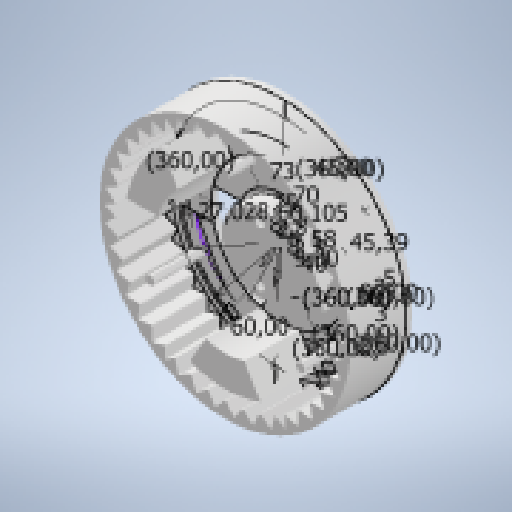
# Autodesk Inventor part: wheel_mold
Saved by Autodesk Inventor 2023 (Build 270158000, 158)
## iProperties
Created: 2026-02-22
Part Number: wheel_mold
Material: Типовые
Document SubType Name: Modeling
Designer: garin
Density: 1 g/cm^3
Appearance: По умолчанию
Author: garin
Autodesk Inventor part; units mm, degrees
ref_plane "YZ Plane" through (0, 0, 0) normal (1, 0, 0) x (0, 1, 0)
ref_plane "XZ Plane" through (0, 0, 0) normal (0, 1, 0) x (-1, 0, 0)
sketch "Эскиз1" plane through (0, 0, 0) normal (0, 0, 1) x (1, 0, 0)
  circle A0 centre (0, 0) radius 35
  circle A1 centre (0, 0) radius 20
  line L0 (0, 0) -> (34.569092, 5.475206) construction
  line L1 (0, 0) -> (35, 0) construction
  line L2 (0, 0) -> (34.569092, -5.475206) construction
  line L3 (34.569092, 5.475206) -> (29.63065, 4.693034) construction
  line L4 (29.63065, 4.693034) -> (19.44159, 4.693034) construction
  line L5 (19.44159, 4.693034) -> (34.683936, 4.693034)
  line L6 (19.44159, -4.693034) -> (34.683936, -4.693034)
  line L7 (13.785082, 14.490394) -> (21.406255, 27.690653) construction
  line L8 (10.751038, 28.007413) -> (5.656509, 19.183428) construction
  line L9 (5.656509, 19.183428) -> (13.277681, 32.383687) construction
  line L10 (-5.656509, 19.183428) -> (-13.277681, 32.383687) construction
  line L11 (-18.879612, 23.314379) -> (-13.785082, 14.490394) construction
  line L12 (-13.785082, 14.490394) -> (-21.406255, 27.690653)
  line L13 (-19.44159, 4.693034) -> (-34.683936, 4.693034)
  line L14 (-29.63065, -4.693034) -> (-19.44159, -4.693034) construction
  line L15 (-19.44159, -4.693034) -> (-34.683936, -4.693034) construction
  line L16 (-13.785082, -14.490394) -> (-21.406255, -27.690653) construction
  line L17 (-10.751038, -28.007413) -> (-5.656509, -19.183428) construction
  line L18 (-5.656509, -19.183428) -> (-13.277681, -32.383687)
  line L19 (5.656509, -19.183428) -> (13.277681, -32.383687) construction
  line L20 (18.879612, -23.314379) -> (13.785082, -14.490394) construction
  line L21 (13.785082, -14.490394) -> (21.406255, -27.690653) construction
  line L22 (0, 0) -> (17.5, 30.310889) construction
  line L23 (0, 0) -> (-17.5, 30.310889) construction
  line L24 (0, 0) -> (-35, 0) construction
  line L25 (0, 0) -> (-17.5, -30.310889) construction
  line L26 (0, 0) -> (17.5, -30.310889) construction
  line L27 (34.683936, 4.693034) -> (29.683936, 4.693034) construction
  line L28 (29.683936, 4.693034) -> (29.683936, -4.693034)
  line L29 (29.683936, 4.693034) -> (29.683936, 1.693034)
  line L30 (29.683936, 1.693034) -> (34.959028, 1.693034)
  line L31 (29.683936, -4.693034) -> (29.683936, -1.693034) construction
  line L32 (29.683936, -1.693034) -> (34.959028, -1.693034)
  line L33 (13.785082, 14.490394) -> (21.406255, 27.690653)
  line L34 (10.751038, 28.007413) -> (5.656509, 19.183428)
  line L35 (13.375758, 26.55356) -> (16.013304, 31.121923)
  line L36 (5.656509, 19.183428) -> (13.277681, 32.383687) construction
  line L37 (10.777681, 28.05356) -> (18.906255, 23.360526)
  line L38 (16.308179, 24.860526) -> (18.945724, 29.428889)
  line L39 (-5.656509, 19.183428) -> (-13.277681, 32.383687) construction
  line L40 (-18.879612, 23.314379) -> (-13.785082, 14.490394)
  line L41 (-16.308179, 24.860526) -> (-18.945724, 29.428889)
  line L42 (-13.785082, 14.490394) -> (-21.406255, 27.690653) construction
  line L43 (-18.906255, 23.360526) -> (-10.777681, 28.05356)
  line L44 (-13.375758, 26.55356) -> (-16.013304, 31.121923)
  line L45 (-19.44159, 4.693034) -> (-34.683936, 4.693034) construction
  line L46 (-29.63065, -4.693034) -> (-19.44159, -4.693034)
  line L47 (-29.683936, -1.693034) -> (-34.959028, -1.693034)
  line L48 (-19.44159, -4.693034) -> (-34.683936, -4.693034) construction
  line L49 (-29.683936, -4.693034) -> (-29.683936, 4.693034)
  line L50 (-29.683936, 1.693034) -> (-34.959028, 1.693034)
  line L51 (-13.785082, -14.490394) -> (-21.406255, -27.690653) construction
  line L52 (-10.751038, -28.007413) -> (-5.656509, -19.183428)
  line L53 (-13.375758, -26.55356) -> (-16.013304, -31.121923)
  line L54 (-5.656509, -19.183428) -> (-13.277681, -32.383687) construction
  line L55 (-10.777681, -28.05356) -> (-18.906255, -23.360526)
  line L56 (-16.308179, -24.860526) -> (-18.945724, -29.428889)
  line L57 (5.656509, -19.183428) -> (13.277681, -32.383687)
  line L58 (18.879612, -23.314379) -> (13.785082, -14.490394)
  line L59 (16.308179, -24.860526) -> (18.945724, -29.428889)
  line L60 (13.785082, -14.490394) -> (21.406255, -27.690653) construction
  line L61 (18.906255, -23.360526) -> (10.777681, -28.05356)
  line L62 (13.375758, -26.55356) -> (16.013304, -31.121923)
  circle A2 centre (0, 0) radius 30.0525
  line L63 (21.406255, 27.690653) -> (20.197155, 25.596431) construction
  line L64 (18.945724, 29.428889) -> (17.445724, 26.830813) construction
  line L65 (17.445724, 26.830813) -> (21.211762, 27.83992)
  line L66 (0, 0) -> (21.211762, 27.83992) construction
  line L67 (21.238374, 23.941121) -> (21.211762, 27.83992)
  line L68 (24.749898, 20.290106) -> (25.338794, 24.144264)
  line L69 (21.46071, 23.742025) -> (25.338794, 24.144264)
  line L70 (27.641356, 16.130756) -> (28.831007, 19.843716)
  line L71 (24.938034, 20.058422) -> (28.831007, 19.843716)
  line L72 (29.840307, 11.567278) -> (31.600908, 15.046017)
  line L73 (27.790578, 15.87229) -> (31.600908, 15.046017)
  line L74 (31.29166, 6.714002) -> (33.579103, 9.871366)
  line L75 (29.946878, 11.288504) -> (33.579103, 9.871366)
  line L76 (31.959055, 1.692518) -> (34.716031, 4.449405)
  line L77 (31.35291, 6.421905) -> (34.716031, 4.449405)
  circle A3 centre (0, 0) radius 32.003841
  line L78 (-14.513304, 28.523847) -> (-13.504197, 32.289885)
  line L79 (-10.114432, 30.363532) -> (-13.504197, 32.289885)
  line L80 (-9.830842, 30.456532) -> (-8.240149, 34.016172)
  line L81 (-5.196798, 31.579093) -> (-8.240149, 34.016172)
  line L82 (14.513764, 28.523613) -> (13.504718, 32.289667)
  line L83 (10.114922, 30.363369) -> (13.504718, 32.289667)
  line L84 (9.831334, 30.456374) -> (8.240698, 34.016039)
  line L85 (5.197307, 31.579009) -> (8.240698, 34.016039)
  line L86 (4.902597, 31.626103) -> (2.770221, 34.890197)
  line L87 (0.149483, 32.003492) -> (2.770221, 34.890197)
  line L88 (-0.148967, 32.003494) -> (-2.769658, 34.890242)
  line L89 (-4.902086, 31.626182) -> (-2.769658, 34.890242)
  line L90 (-31.959028, 1.693034) -> (-34.715959, 4.449965)
  line L91 (-31.352806, 6.422411) -> (-34.715959, 4.449965)
  line L92 (-31.291552, 6.714507) -> (-33.578943, 9.871908)
  line L93 (-29.946696, 11.288988) -> (-33.578943, 9.871908)
  line L94 (-17.445291, 26.831095) -> (-21.211313, 27.840262)
  line L95 (-21.237988, 23.941464) -> (-21.211313, 27.840262)
  line L96 (-21.460327, 23.742372) -> (-25.338405, 24.144673)
  line L97 (-24.749571, 20.290505) -> (-25.338405, 24.144673)
  line L98 (-24.93771, 20.058825) -> (-28.830687, 19.844181)
  line L99 (-27.641095, 16.131202) -> (-28.830687, 19.844181)
  line L100 (-27.790322, 15.872738) -> (-31.600665, 15.046527)
  line L101 (-29.84012, 11.56776) -> (-31.600665, 15.046527)
  line L102 (-17.445724, -26.830813) -> (-21.211762, -27.83992)
  line L103 (-21.238374, -23.941121) -> (-21.211762, -27.83992)
  line L104 (-21.46071, -23.742025) -> (-25.338794, -24.144264)
  line L105 (-24.749898, -20.290106) -> (-25.338794, -24.144264)
  line L106 (-31.959055, -1.692518) -> (-34.716031, -4.449405)
  line L107 (-31.35291, -6.421905) -> (-34.716031, -4.449405)
  line L108 (-31.29166, -6.714002) -> (-33.579103, -9.871366)
  line L109 (-29.946878, -11.288504) -> (-33.579103, -9.871366)
  line L110 (-29.840307, -11.567278) -> (-31.600908, -15.046017)
  line L111 (-27.790578, -15.87229) -> (-31.600908, -15.046017)
  line L112 (-27.641356, -16.130756) -> (-28.831007, -19.843716)
  line L113 (-24.938034, -20.058422) -> (-28.831007, -19.843716)
  line L114 (14.513304, -28.523847) -> (13.504197, -32.289885)
  line L115 (10.114432, -30.363532) -> (13.504197, -32.289885)
  line L116 (9.830842, -30.456532) -> (8.240149, -34.016172)
  line L117 (5.196798, -31.579093) -> (8.240149, -34.016172)
  line L118 (-14.513764, -28.523613) -> (-13.504718, -32.289667)
  line L119 (-10.114922, -30.363369) -> (-13.504718, -32.289667)
  line L120 (-9.831334, -30.456374) -> (-8.240698, -34.016039)
  line L121 (-5.197307, -31.579009) -> (-8.240698, -34.016039)
  line L122 (-4.902597, -31.626103) -> (-2.770221, -34.890197)
  line L123 (-0.149483, -32.003492) -> (-2.770221, -34.890197)
  line L124 (0.148967, -32.003494) -> (2.769658, -34.890242)
  line L125 (4.902086, -31.626182) -> (2.769658, -34.890242)
  line L126 (31.959028, -1.693034) -> (34.715959, -4.449965)
  line L127 (31.352806, -6.422411) -> (34.715959, -4.449965)
  line L128 (31.291552, -6.714507) -> (33.578943, -9.871908)
  line L129 (29.946696, -11.288988) -> (33.578943, -9.871908)
  line L130 (17.445291, -26.831095) -> (21.211313, -27.840262)
  line L131 (21.237988, -23.941464) -> (21.211313, -27.840262)
  line L132 (21.460327, -23.742372) -> (25.338405, -24.144673)
  line L133 (24.749571, -20.290505) -> (25.338405, -24.144673)
  line L134 (24.93771, -20.058825) -> (28.830687, -19.844181)
  line L135 (27.641095, -16.131202) -> (28.830687, -19.844181)
  line L136 (27.790322, -15.872738) -> (31.600665, -15.046527)
  line L137 (29.84012, -11.56776) -> (31.600665, -15.046527)
  circle A4 centre (0, 0) radius 11
  line L138 (0, 0) -> (0, 8) construction
  circle A5 centre (0, 8) radius 1.25
  circle A6 centre (0, -8) radius 1.25
  line L139 (0, 0) -> (8, 0) construction
  circle A7 centre (8, 0) radius 1.25
  circle A8 centre (-8, 0) radius 1.25
  circle A9 centre (0, 0) radius 12.5
  circle A10 centre (0, 0) radius 36.5
  arc A11 (-13.785082, 14.490394) -> (-19.44159, 4.693034) centre (0, 0) ccw
  line L140 (-26.974922, 1.693034) -> (-26.974922, -1.693034)
  line L141 (-29.683936, 1.693034) -> (-26.974922, 1.693034)
  line L142 (-26.974922, -1.693034) -> (-29.683936, -1.693034)
  line L143 (-12.021251, -24.207485) -> (-13.375758, -26.55356)
  line L144 (-16.308179, -24.860526) -> (-14.953671, -22.514451)
  line L145 (-14.953671, -22.514451) -> (-12.021251, -24.207485)
  line L146 (14.953671, -22.514451) -> (16.308179, -24.860526)
  line L147 (13.375758, -26.55356) -> (12.021251, -24.207485)
  line L148 (12.021251, -24.207485) -> (14.953671, -22.514451)
  line L149 (26.974922, 1.693034) -> (29.683936, 1.693034)
  line L150 (29.683936, -1.693034) -> (26.974922, -1.693034)
  line L151 (26.974922, -1.693034) -> (26.974922, 1.693034)
  line L152 (12.021251, 24.207485) -> (13.375758, 26.55356)
  line L153 (16.308179, 24.860526) -> (14.953671, 22.514451)
  line L154 (14.953671, 22.514451) -> (12.021251, 24.207485)
  line L155 (-14.953671, 22.514451) -> (-16.308179, 24.860526)
  line L156 (-13.375758, 26.55356) -> (-12.021251, 24.207485)
  line L157 (-12.021251, 24.207485) -> (-14.953671, 22.514451)
  line L158 (31.959055, 1.692518) -> (35, 0)
  line L159 (31.959028, -1.693034) -> (35, 0)
  line L160 (14.513764, 28.523613) -> (17.5, 30.310889)
  line L161 (17.445724, 26.830813) -> (17.5, 30.310889)
  line L162 (-17.445291, 26.831095) -> (-17.5, 30.310889)
  line L163 (-14.513304, 28.523847) -> (-17.5, 30.310889)
  line L164 (-31.959055, -1.692518) -> (-35, 0)
  line L165 (-31.959028, 1.693034) -> (-35, 0)
  line L166 (-14.513764, -28.523613) -> (-17.5, -30.310889)
  line L167 (-17.445724, -26.830813) -> (-17.5, -30.310889)
  line L168 (17.445291, -26.831095) -> (17.5, -30.310889)
  line L169 (14.513304, -28.523847) -> (17.5, -30.310889)
  line L170 (19.44159, -4.693034) -> (29.683936, -4.693034)
  line L171 (18.906255, -23.360526) -> (13.785082, -14.490394)
  line L172 (16.345668, -18.92546) -> (24.562763, -4.693034)
  arc A12 (16.345668, -18.92546) -> (24.562763, -4.693034) centre (3.305498, -1.90843) ccw
  line L173 (24.562763, 4.693034) -> (16.345668, 18.92546)
  arc A13 (24.562763, 4.693034) -> (16.345668, 18.92546) centre (3.305498, 1.90843) ccw
  line L174 (8.217095, 23.618494) -> (-8.217095, 23.618494)
  arc A14 (8.217095, 23.618494) -> (-8.217095, 23.618494) centre (0, 3.81686) ccw
  line L175 (-16.345668, 18.92546) -> (-24.562763, 4.693034)
  arc A15 (-16.345668, 18.92546) -> (-24.562763, 4.693034) centre (-3.305498, 1.90843) ccw
  line L176 (-24.562763, -4.693034) -> (-16.345668, -18.92546)
  arc A16 (-24.562763, -4.693034) -> (-16.345668, -18.92546) centre (-3.305498, -1.90843) ccw
  line L177 (-8.217095, -23.618494) -> (8.217095, -23.618494)
  arc A17 (-8.217095, -23.618494) -> (8.217095, -23.618494) centre (0, -3.81686) ccw
  circle A18 centre (21.872108, -12.627867) radius 1.25
  circle A19 centre (21.872108, 12.627867) radius 1.25
  circle A20 centre (0, 25.255735) radius 1.25
  circle A21 centre (-21.872108, 12.627867) radius 1.25
  circle A22 centre (-21.872108, -12.627867) radius 1.25
  circle A23 centre (0, -25.255735) radius 1.25
  circle A24 centre (0, 0) radius 29
  line L178 (-10.244587, -27.130213) -> (-1.728498, -12.379915)
  line L179 (-10.244587, -27.130213) -> (6.78759, -27.130213) construction
  line L180 (-24.562763, 4.693034) -> (-11.58557, 4.693034)
  line L181 (28.617747, -4.693034) -> (11.58557, -4.693034)
  line L182 (8.217095, 23.618494) -> (1.728498, 12.379915)
  point P0 (31.959028, -1.693034)
  point P1 (17.445996, -26.831283)
  point P2 (14.513304, -28.523847)
  point P3 (-14.513575, -28.524317)
  point P4 (-31.959571, -1.693034)
  point P5 (-31.959028, 1.693034)
  point P6 (-17.445996, 26.831283)
  point P7 (-14.513304, 28.523847)
  point P8 (14.513575, 28.524317)
  point P9 (31.959571, 1.693034)
  point P10 (10.778409, -28.05314)
  point P11 (18.905527, -23.360946)
  point P12 (29.683936, -4.692194)
  point P13 (29.683936, 4.692194)
  point P14 (18.905527, 23.360946)
  point P15 (10.778409, 28.05314)
  point P16 (-10.778409, 28.05314)
  point P17 (-18.905527, 23.360946)
  point P18 (-29.683936, 4.692194)
  point P19 (-29.683936, -4.692194)
  point P20 (-18.905527, -23.360946)
  point P21 (-10.778409, -28.05314)
  point P22 (10.777615, -28.053445)
  point P23 (-10.777615, -28.053445)
  point P24 (29.683803, 4.693034)
  point P25 (18.906188, 23.360411)
  point P26 (-18.906188, 23.360411)
  point P27 (-29.683803, 4.693034)
  point P28 (-14.513304, -28.523847)
  point P29 (17.445724, -26.830813)
  point P30 (31.959028, 1.693034)
  point P31 (14.513304, 28.523847)
  point P32 (-17.445724, 26.830813)
  point P33 (-31.959028, -1.693034)
  point P34 (-35, 0)
  point P35 (-35, 0)
  point P36 (-31.959028, 1.693034)
  point P37 (-14.513304, 28.523847)
  point P38 (17.445724, 26.830813)
  point P39 (35, 0)
  point P40 (35, 0)
  point P41 (31.959028, -1.693034)
  point P42 (14.513304, -28.523847)
  point P43 (-18.37316, 22.437179)
  point P44 (-28.617747, 4.693034)
  point P45 (28.617747, 4.693034)
  point P46 (18.37316, 22.437179)
  point P47 (-10.244587, -27.130213)
  point P48 (10.244587, -27.130213)
  point P49 (1.728498, 12.379915)
  dimension "d10" = 70
  dimension "d11" = 40
  dimension "d57" = 58
  dimension "d12" = 9
  dimension "d13" = 5
  dimension "d14" = 360
  dimension "d15" = 360
  dimension "d16" = 5
  dimension "d17" = 90
  dimension "d18" = 3
  dimension "d19" = 3
  dimension "d20" = 360
  dimension "d21" = 60.105
  dimension "d22" = 3
  dimension "d23" = 45
  dimension "d24" = 45.392
  dimension "d25" = 360
  dimension "d26" = 22
  dimension "d27" = 8
  dimension "d28" = 2.5
  dimension "d29" = 8
  dimension "d30" = 2.5
  dimension "d31" = 25
  dimension "d32" = 73
  dimension "d39" = 27.028
  dimension "d42" = 360
  dimension "d46" = 360
  dimension "d50" = 360
  dimension "d52" = 2.5
  dimension "d55" = 360
  dimension "d58" = 60
  constraints: 366 end point, 43 point on line, 21 centre point, 17 point on circle, 10 coincident, 9 symmetric about line, 5 horizontal, 2 collinear, 2 equal length, 2 midpoint, 2 perpendicular, 2 vertical, 515 other
  measures "d12" angle of L1 L0
  measures "d13" distance of L0.end L4.start
  measures "d16" distance of L5.end L29.start
  measures "d17" angle of L28 L27
  measures "d18" distance of L29.start L29.end
  measures "d19" distance of L28.end L31.end
  measures "d21" diameter of A2
  measures "d22" distance of L38.end L64.end
  measures "d23" angle of L65 L64
  measures "d26" diameter of A4
  measures "d27" distance of L139.start L138.end
  measures "d28" diameter of A5
  measures "d29" distance of L139.start L139.end
  measures "d30" diameter of A7
  measures "d31" diameter of A9
  measures "d32" diameter of A10
  measures "d39" distance of A11.centre L140.start
  measures "d52" diameter of A18
  measures "d58" angle of L179 L178
ref_plane "РабПлоскость1" through (-29.683803, -23.360411, -2) normal (0, 0, -1) x (0, 1, 0)
extrude "Выдавливание1" add sketch "Эскиз1" along normal blind 18 from surface at -2 contours L158 L30 A0 | A0 L32 L159 | L30 L76 A0 | A0 L126 L32 | L77 L5 A0 | A0 L6 L127 | L5 L77 A3 L74 A0 | A0 L128 A3 L127 L6 | L75 A3 L72 A0 | A0 L137 A3 L129 | L5 A13 A19 L33 A24 | L73 A3 L70 A0 | A0 L135 A3 L136 | L5 A1 L33 L173 | L173 A13 A19 | L71 A3 L68 A0 | A0 L133 A3 L134 | A19 A13 | A13 A19 | L67 A0 L33 | L33 A0 L69 A3 L67 | L161 A0 L38 | L38 A0 L65 | A18 A12 | A12 A18 | L130 A0 L59 | L59 A0 L168 | A0 L131 A3 L132 | L82 A0 L35 | L35 A0 L160 | L169 A0 L62 | L62 A0 L114 | A3 L84 A0 L83 | L57 L177 L18 A1 | A24 L18 A17 A23 L57 | A0 L57 L115 | A1 L13 L175 L12 | L85 A3 L86 A0 | A17 A23 L177 | L57 A0 L116 A3 L115 | A15 A21 L13 A24 L12 | L175 A15 A21 | A20 A14 | A14 A20 | L87 A3 L88 A0 | L163 A0 L44 | L44 A0 L78 | A23 A17 | A17 A23 | L119 A3 L120 A0 L18 | L18 A0 L119 | L118 A0 L53 | L53 A0 L166 | A0 L125 A3 L117 | A21 A15 | A15 A21 | L89 A3 L81 A0 | L79 A0 L80 A3 | L94 A0 L41 | L41 A0 L162 | L167 A0 L56 | L56 A0 L102 | A0 L123 A3 L124 | L95 L12 A0 | A22 A16 | A16 A22 | L121 A3 L122 A0 | L103 A0 L104 A3 | L95 A3 L96 A0 L12 | A0 L113 A3 L105 | L91 A0 L13 | L13 A0 L92 A3 L91 | L165 A0 L50 | L50 A0 L90 | L97 A3 L98 A0 | A0 L111 A3 L112 | L106 A0 L47 | L47 A0 L164 | L99 A3 L100 A0 | A0 L109 A3 L110 | A3 L108 A0 L107 | A0 L101 A3 L93 | A4 | A7 | A8 | A10
extrude "Выдавливание2" add sketch "Эскиз1" against normal blind 2 contours L158 L30 A0 | L159 A3 L158 | A0 L32 L159 | L30 L76 A0 | A0 L126 L32 | A3 L32 A2 L30 | A3 L5 L77 L76 | L30 A2 L5 A3 | A3 L6 A2 L32 | L126 L127 L6 A3 | L77 L5 A0 | A0 L6 L127 | A2 L32 L28 L30 | L30 L28 A2 | A3 L77 L5 | L5 A2 L33 A3 | A2 L28 L32 | A3 L59 A2 L6 | L6 L127 A3 | L5 L77 A3 L74 A0 | A0 L128 A3 L127 L6 | L149 A24 L5 L28 | L28 L150 A24 L149 | L5 A24 L33 A2 | L28 L6 A24 L150 | A2 L171 L58 A24 L6 | L75 A3 L72 A0 | L74 A3 L75 | L129 A3 L128 | A0 L137 A3 L129 | A24 L150 L151 L149 | L149 L151 L150 A24 L6 A1 L5 | L5 A13 A19 L33 A24 | A2 L38 A3 L33 | L33 A24 L153 L37 | L37 L38 A2 | A24 L58 A12 A18 L6 | A2 L59 L61 | L61 L146 A24 L58 L171 | L73 A3 L70 A0 | L72 A3 L73 | A0 L135 A3 L136 | L136 A3 L137 | L5 A1 L33 L173 | L173 A13 A19 | L33 A1 L34 A24 L152 L154 L153 | A3 L65 L67 L33 | L33 L67 A3 | L153 A24 L152 L37 | L37 L35 A2 L38 | A2 L35 A3 L38 | L172 L58 A1 L6 | A12 A18 L172 | A24 L146 L148 L147 L57 A1 L58 | L59 A2 L62 L61 | L61 L147 A24 L146 | L59 A3 L62 A2 | L71 A3 L68 A0 | L70 A3 L71 | A0 L133 A3 L134 | L134 A3 L135 | A19 A13 | A13 A19 | L153 L154 L152 A24 | L67 A0 L33 | L33 A0 L69 A3 L67 | L161 A0 L38 | L38 A0 L65 | A3 L160 L161 | L37 A2 L35 | L152 A24 L156 L43 A2 L37 | A2 L44 A3 L35 | A1 L178 A9 L181 | A18 A12 | A12 A18 | A24 L147 L148 L146 | L62 A2 L61 | L61 L57 A24 L147 | L130 A0 L59 | L168 L169 A3 | A3 L131 L130 | L59 A0 L168 | L62 A3 L57 A2 | L68 A3 L69 | A0 L131 A3 L132 | L132 A3 L133 | L82 A0 L35 | A3 L83 L82 | L35 A0 L160 | A9 | A2 L18 A24 L57 | L57 A3 L18 A2 | L169 A0 L62 | L114 L115 L57 A3 | L62 A0 L114 | L182 A9 L180 A1 | L174 A14 A20 | A1 L12 A24 L155 L157 L156 L34 | A3 L84 A0 L83 | L43 L44 A2 | L57 L177 L18 A1 | A24 L18 A17 A23 L57 | L57 L115 A3 | L55 L143 A24 L18 | A2 L53 L55 | L18 A3 L53 A2 | A0 L57 L115 | A1 L13 L175 L12 | A24 L155 L43 L156 | L156 L157 L155 A24 | A3 L85 L84 | L85 A3 L86 A0 | L43 L41 A2 L44 | A2 L41 A3 L44 | L176 A16 A22 | L18 A24 L143 L145 L144 L46 A1 | A17 A23 L177 | L57 A0 L116 A3 L115 | A3 L119 L18 | L18 L119 L118 A3 | L53 A2 L56 L55 | L55 L144 A24 L143 | L53 A3 L56 A2 | A1 L46 A24 L142 L140 L141 L13 | A15 A21 L13 A24 L12 | L175 A15 A21 | A20 A14 | A14 A20 | A24 L12 L43 L155 | L87 A3 L88 A0 | L86 A3 L87 | L43 A2 L41 | L163 A0 L44 | L78 L79 A3 | L44 A0 L78 | A3 L162 L163 | A2 L12 A3 L41 | A23 A17 | A17 A23 | A24 L144 L145 L143 | L116 L117 A3 | L119 A3 L120 A0 L18 | L18 A0 L119 | L118 A0 L53 | L166 L167 A3 | L53 A0 L166 | L56 A2 L55 | L55 A2 L49 L142 A24 L144 | L56 A3 L47 A2 | A0 L125 A3 L117 | A24 L13 A2 L12 | A21 A15 | A15 A21 | L89 A3 L81 A0 | L88 A3 L89 | A2 L13 A3 L12 | L79 A0 L80 A3 | L94 A0 L41 | A3 L12 L95 L94 | L41 A0 L162 | L167 A0 L56 | L102 L103 A3 | L56 A0 L102 | A3 L121 L120 | A0 L123 A3 L124 | L124 A3 L125 | A24 L141 L49 L13 | L81 A3 L80 | A3 L95 L12 | A2 L50 A3 L13 | L49 L50 A2 | L95 L12 A0 | A22 A16 | A16 A22 | L121 A3 L122 A0 | L103 A0 L104 A3 | A2 L47 L49 | L122 A3 L123 | A24 L142 L49 L141 | L141 L140 L142 A24 | L95 A3 L96 A0 L12 | A3 L90 L91 L13 | L13 L91 A3 | L49 L47 A2 L50 | A2 L47 A3 L50 | L104 L105 A3 | A0 L113 A3 L105 | A3 L97 L96 | L91 A0 L13 | L13 A0 L92 A3 L91 | L165 A0 L50 | L50 A0 L90 | A3 L164 L165 | L97 A3 L98 A0 | A0 L111 A3 L112 | L112 A3 L113 | L106 A0 L47 | A3 L107 L106 | L47 A0 L164 | L92 L93 A3 | L99 A3 L100 A0 | L98 A3 L99 | A0 L109 A3 L110 | L110 A3 L111 | A3 L108 A0 L107 | A0 L101 A3 L93 | L100 A3 L101 | L108 A3 L109 | A4 | A5 | A6 | A7 | A8 | A10
extrude "Выдавливание3" cut sketch "Эскиз1" against normal blind 10 from surface at 16 contours A4 | A7 | A8
